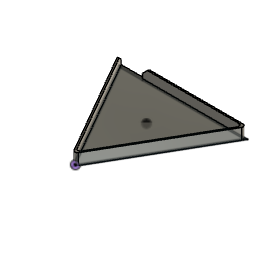
Pill Counter (Autodesk Fusion 360 design; units mm, degrees)
Autodesk Fusion 360 part; units mm, degrees
sketch "Sketch1" plane through (0, 0, 0) normal (0, 0, 1) x (1, 0, 0)
  line L0 (-50, 86.6025) -> (0, 0)
  line L1 (0, 0) -> (50, 86.6025)
  line L2 (50, 86.6025) -> (-50, 86.6025)
  line L3 (52.0785, 87.8025) -> (-52.0785, 87.8025)
  line L4 (-52.0785, 87.8025) -> (0, -2.4)
  line L5 (0, -2.4) -> (52.0785, 87.8025)
  line L6 (-32.0785, 86.6025) -> (-32.0785, 87.8025)
  line L7 (-50, 86.6025) -> (-50.6928, 87.8025)
  point P0 (0, 57.735)
  dimension "d1" = 100
  dimension "d2" = 1.2
  dimension "d11" = 20
  constraint horizontal L2
  constraint coincident L0.end L1.start
  constraint coincident L2 L6.start
  constraint coincident L3 L6.end
  constraint perpendicular L3 L6
  constraint coincident L3 L7.end
  constraint parallel L0 L7
  measures "d1" distance of L0.start L1.end
  measures "d11" distance of L3.end L6
extrude "Extrude1" add sketch "Sketch1" along normal blind 1.2 contours L0 L1 L2 | L2 L3 L6 L7
extrude "Extrude2" add sketch "Sketch1" along normal blind 9 contours L0 L1 L2 L3 L4 L5 L6 L7
fillet "Fillet1" radius 2 2 edges at (50, 86.6025, 5.1) (0, 0, 5.1)
fillet "Fillet1" radius 2 2 edges at (52.0785, 87.8025, 4.5) (0, -2.4, 4.5)
chamfer "Chamfer1" distance 4 angle 45 2 edges at (-51.3856, 87.8025, 9) (-32.0785, 87.2025, 9) tangent chain off
named bodies: "Pill Counter"
